Autodesk Inventor part; units mm, degrees
(part 2 of 2)
sketch "Sketch9" plane through (0, 1.905, 0) normal (0, -1, 0) x (1, 0, 0)
  line L0 (13.8812, 7.3449) -> (13.8812, -7.0624) construction
  line L1 (13.8812, -7.0624) -> (-14.7275, -7.0624) construction
  line L2 (-14.7275, -7.0624) -> (-14.7275, 7.3449) construction
  line L3 (-14.7275, 7.3449) -> (13.8812, 7.3449) construction
  line L4 (-0.4231, 7.3449) -> (14.5824, 7.3449) construction
  circle A0 centre (0, 0) radius 12.7 projected
  line L5 (0, 12.7) -> (0, -12.7)
  line L6 (12.7, 0) -> (-12.7, 0)
  line L7 (-0.0381, 0.5025) -> (-4.1246, 4.589)
  line L8 (0, 0.4644) -> (7.62, 0.4644) construction
  line L9 (-5.3066, 4.6096) -> (-10.2786, -0.0268)
  line L10 (-4.7057, 5.17) -> (2.0926, 5.17) construction
  line L11 (0.0876, 0.5025) -> (4.0727, 4.4876)
  line L12 (8.6079, 2.3126) -> (4.6852, 4.5688)
  line L13 (0.9377, 0.4595) -> (4.1978, 3.6576)
  line L14 (4.7324, 3.7704) -> (8.6079, 2.3126)
  line L15 (1, 0.3071) -> (7.5359, 0.3071)
  arc A1 (7.5359, 0.3071) -> (9.1739, 0.8317) centre (7.1665, 4.28) ccw
  arc A2 (9.1739, 0.8317) -> (8.5726, 0.2974) centre (12.9474, -4.0204) ccw
  arc A3 (8.5726, 0.2974) -> (8.6079, 0.1777) centre (8.6109, 0.2436) ccw
  arc A4 (10.1384, 0) -> (8.6079, 0.1777) centre (8.4908, -7.5095) ccw
  line L16 (0, -0.5397) -> (0.0115, -0.5512)
  line L17 (-4.7229, 4.1832) -> (-4.6451, 4.2557)
  line L18 (-4.5584, 4.169) -> (-0.8385, 0.4491)
  line L19 (-0.9013, 0.2974) -> (-8.6642, 0.2974)
  line L20 (-8.7249, 0.4513) -> (-4.7348, 4.1721)
  arc A5 (-4.1246, 4.589) -> (-5.3066, 4.6096) centre (-4.7263, 3.9873) ccw
  arc A6 (4.6852, 4.5688) -> (4.0727, 4.4876) centre (4.432, 4.1284) ccw
  arc A7 (4.7324, 3.7704) -> (4.1978, 3.6576) centre (4.5536, 3.2949) ccw
  arc A8 (-4.5584, 4.169) -> (-4.7348, 4.1721) centre (-4.6482, 4.0792) ccw
  arc A9 (-8.7249, 0.4513) -> (-8.6642, 0.2974) centre (-8.6642, 0.3863) ccw
  arc A10 (-0.9013, 0.2974) -> (-0.8385, 0.4491) centre (-0.9013, 0.3863) ccw
  arc A11 (0.9377, 0.4595) -> (1, 0.3071) centre (1, 0.396) ccw
  arc A12 (-0.0381, 0.5025) -> (0.0876, 0.5025) centre (0.0247, 0.5653) ccw
  line L21 (-0.0381, -0.5025) -> (-4.1246, -4.589)
  line L22 (-5.3066, -4.6096) -> (-10.2786, 0.0268)
  line L23 (0.0876, -0.5025) -> (4.0727, -4.4876)
  line L24 (8.6079, -2.3126) -> (4.6852, -4.5688)
  line L25 (0.9377, -0.4595) -> (4.1978, -3.6576)
  line L26 (4.7324, -3.7704) -> (8.6079, -2.3126)
  line L27 (1, -0.3071) -> (7.5359, -0.3071)
  arc A13 (9.1739, -0.8317) -> (7.5359, -0.3071) centre (7.1665, -4.28) ccw
  arc A14 (8.5726, -0.2974) -> (9.1739, -0.8317) centre (12.9474, 4.0204) ccw
  arc A15 (8.6079, -0.1777) -> (8.5726, -0.2974) centre (8.6109, -0.2436) ccw
  arc A16 (8.6079, -0.1777) -> (10.1384, 0) centre (8.4908, 7.5095) ccw
  line L28 (-4.5584, -4.169) -> (-0.8385, -0.4491)
  line L29 (-0.9013, -0.2974) -> (-8.6642, -0.2974)
  line L30 (-8.7249, -0.4513) -> (-4.7348, -4.1721)
  arc A17 (-5.3066, -4.6096) -> (-4.1246, -4.589) centre (-4.7263, -3.9873) ccw
  arc A18 (4.0727, -4.4876) -> (4.6852, -4.5688) centre (4.432, -4.1284) ccw
  arc A19 (4.1978, -3.6576) -> (4.7324, -3.7704) centre (4.5536, -3.2949) ccw
  arc A20 (-4.7348, -4.1721) -> (-4.5584, -4.169) centre (-4.6482, -4.0792) ccw
  arc A21 (-8.6642, -0.2974) -> (-8.7249, -0.4513) centre (-8.6642, -0.3863) ccw
  arc A22 (-0.8385, -0.4491) -> (-0.9013, -0.2974) centre (-0.9013, -0.3863) ccw
  arc A23 (1, -0.3071) -> (0.9377, -0.4595) centre (1, -0.396) ccw
  arc A24 (0.0876, -0.5025) -> (-0.0381, -0.5025) centre (0.0247, -0.5653) ccw
  point P0 (5.4129, 5.8278)
  point P1 (-10.2498, 0)
  dimension "d273" = 135
  dimension "d274" = 7.62
  dimension "d275" = 137
  dimension "d277" = 6.6548
  dimension "d298" = 0.8509
  dimension "d299" = 0.508
  dimension "d300" = 0.508
  dimension "d301" = 0.127
  dimension "d302" = 0.0889
  dimension "d304" = 0.0889
  constraints: 54 end point, 54 point on circle, 35 symmetric about line, 24 centre point, 16 tangent, 9 point on line, 6 horizontal, 2 equal radius, 1 equal length, 1 midpoint, 1 vertical, 14 other
  measures "d273" angle of L8 L7
  measures "d274" distance of L10.start L9.end
  measures "d275" angle of L9 L10
  measures "d277" distance of L8.start L10.start
  measures "d298" radius of A5
  measures "d299" radius of A6
  measures "d300" radius of A7
  measures "d301" radius of A8
  measures "d302" radius of A9
  measures "d304" radius of A12
extrude "Extrusion8" add sketch "Sketch9" along normal blind 1.905 contours A16 A15 A14 A13 L27 A23 L25 A19 L26 L24 A18 L23 A24 L5 L6 | L6 L5 A12 L11 A6 L12 L14 A7 L13 A11 L15 A1 A2 A3 A4 | L5 L6 L9 A5 L7 A12 | L5 A24 L21 A17 L22 L6
body "Solid1"
